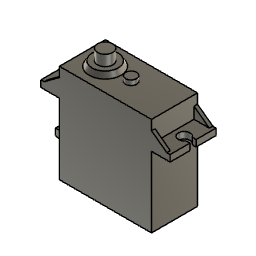
GWSservo v6 (Autodesk Fusion 360 design; units mm, degrees)
Autodesk Fusion 360 part; units mm, degrees
sketch "スケッチ1" plane through (0, 0, 0) normal (0, 1, 0) x (1, 0, 0)
  line L0 (-28.35, -21.75) -> (0, -21.75)
  line L1 (0, -21.75) -> (0, 0)
  line L2 (0, 0) -> (-28.35, 0)
  line L3 (-28.35, 0) -> (-28.35, -21.75)
  dimension "d1" = 28.35
  dimension "d2" = 21.75
  constraint horizontal L0
  constraint vertical L1
  constraint horizontal L2
  constraint vertical L3
  constraint coincident L1.end L2.start
  measures "d1" distance of L0.start L0.end
  measures "d2" distance of L0.start L2.end
extrude "押し出し1" add sketch "スケッチ1" along normal blind 14.15 makes body 1
sketch "スケッチ2" plane through (0, 0, 0) normal (0, -1, 0) x (1, 0, 0)
  line L0 (-28.35, 21.75) -> (-28.35, 0)
  line L1 (-28.35, 0) -> (0, 0)
  line L2 (0, 0) -> (0, 21.75)
  line L3 (0, 21.75) -> (-28.35, 21.75)
  line L4 (-34.075, 21.75) -> (5.725, 21.75)
  line L5 (5.725, 21.75) -> (5.725, 23.75)
  line L6 (0, 27.25) -> (0, 30.25)
  line L7 (0, 30.25) -> (-28.35, 30.25)
  line L8 (-28.35, 30.25) -> (-28.35, 27.25)
  line L9 (-34.075, 23.75) -> (-34.075, 21.75)
  line L10 (-28.35, 27.25) -> (-33.075, 23.75)
  line L11 (-33.075, 23.75) -> (-34.075, 23.75)
  line L12 (0, 27.25) -> (4.725, 23.75)
  line L13 (4.725, 23.75) -> (5.725, 23.75)
  dimension "d5" = 2
  dimension "d6" = 30.25
  dimension "d7" = 5.5
  dimension "d8" = 39.8
  dimension "d9" = 1
  dimension "d15" = 3
  dimension "d16" = 28.35
  dimension "d73" = 28.35
  constraint perpendicular L4 L5
  constraint perpendicular L4 L6
  constraint perpendicular L7 L8
  constraint vertical L9
  constraint midpoint L3 L4
  constraint collinear L3 L4
  constraint equal L5 L9
  constraint equal L6 L8
  constraint vertical L8
  constraint collinear L0 L8
  constraint equal L10 L12
  constraint equal L11 L13
  constraint horizontal L13
  measures "d5" distance of L4.start L9.start
  measures "d6" distance of L1 L7
  measures "d7" distance of L4 L8.end
  measures "d8" distance of L5.end L9.start
  measures "d9" distance of L5.end L12.end
  measures "d15" distance of L6.start L7
  measures "d16" distance of L6.end L7.end
  measures "d73" distance of L0 L2
extrude "押し出し2" add sketch "スケッチ2" against normal blind 14.15 contours L3 L4 L5 L6 L7 L8 L9 L10 L11 L12 L13 bodies 1
ref_plane "作業平面1" through (0, 7.075, 0) normal (0, 1, 0) x (0, 0, 1)
sketch "スケッチ3" plane through (0, 7.075, 0) normal (0, 1, 0) x (1, 0, 0)
  line L0 (0, -27.25) -> (4.725, -23.75)
  line L1 (0, -23.75) -> (0, -27.25)
  line L2 (4.725, -23.75) -> (0, -23.75)
  line L3 (-14.175, -35.735) -> (-14.175, -20.735) construction
  line L4 (-33.075, -23.75) -> (-28.35, -23.75)
  line L5 (-28.35, -27.25) -> (-33.075, -23.75)
  line L6 (-28.35, -23.75) -> (-28.35, -27.25)
  line L7 (-28.35, -21.75) -> (-28.35, 0)
  line L8 (-28.35, 0) -> (0, 0)
  line L9 (0, 0) -> (0, -21.75)
  line L10 (0, -21.75) -> (5.725, -21.75)
  line L11 (5.725, -21.75) -> (5.725, -23.75)
  line L12 (5.725, -23.75) -> (4.725, -23.75)
  line L13 (4.725, -23.75) -> (0, -27.25)
  line L14 (0, -27.25) -> (0, -30.25)
  line L15 (0, -30.25) -> (-28.35, -30.25)
  line L16 (-28.35, -30.25) -> (-28.35, -27.25)
  line L17 (-28.35, -27.25) -> (-33.075, -23.75)
  line L18 (-33.075, -23.75) -> (-34.075, -23.75)
  line L19 (-34.075, -23.75) -> (-34.075, -21.75)
  line L20 (-34.075, -21.75) -> (-28.35, -21.75)
  dimension "d70" = 28.35
  dimension "d71" = 14.175
  dimension "d72" = 2
  constraint coincident L0.end L2.start
  constraint horizontal L2
  constraint vertical L1
  constraint vertical L3
  constraint symmetric L1.start L3 L4.end
  constraint symmetric L0.end L3 L4.start
  constraint symmetric L0.start L3 L5.start
  constraint collinear L1 L14
  constraint coincident L0.start L1.end
  measures "d70" distance of L14.end L15.end
  measures "d71" distance of L3 L15.end
  measures "d72" distance of L2 L10
extrude "押し出し3" cut sketch "スケッチ3" along normal mid plane 12 contours L0 L1 L2 L13 | L4 L5 L6 L17 bodies 1
sketch "スケッチ4" plane through (0, 0, 30.25) normal (0, 0, 1) x (-1, 0, 0)
  line L0 (28.35, 0) -> (0, 0)
  line L1 (0, 0) -> (0, -14.15)
  line L2 (0, -14.15) -> (28.35, -14.15)
  line L3 (28.35, -14.15) -> (28.35, 0)
  circle A0 centre (13.35, -7.075) radius 1.7
  circle A1 centre (21.35, -7.075) radius 4.9
  line L4 (28.35, -7.075) -> (-4.65, -7.075) construction
  dimension "d17" = 3.4
  dimension "d18" = 9.8
  dimension "d19" = 15
  dimension "d20" = 7
  dimension "d75" = 14.15
  dimension "d76" = 7.075
  constraint perpendicular L1 L4
  constraint midpoint L3 L4.start
  constraint coincident A0.centre L4
  constraint coincident A1.centre L4
  measures "d17" diameter of A0
  measures "d18" diameter of A1
  measures "d19" distance of A0.centre L4.start
  measures "d20" distance of A1.centre L4.start
  measures "d75" distance of L0 L2
  measures "d76" distance of L0 A1.centre
extrude "押し出し4" add sketch "スケッチ4" along normal blind 1.5 contours A0 bodies 1
ref_plane "作業平面2" through (-14.175, 7.075, 31.75) normal (0, 0, 1) x (1, 0, 0)
sketch "スケッチ5" plane through (-14, 7, 31.75) normal (0, 0, 1) x (1, 0, 0)
  circle A0 centre (-7.35, 0.075) radius 4
  line L0 (-14.35, -7) -> (-14.35, 7.15)
  line L1 (14, -7) -> (-14.35, -7)
  dimension "d24" = 8
  dimension "d25" = 7
  dimension "d74" = 7.075
  dimension "d77" = 14.15
  measures "d24" diameter of A0
  measures "d25" distance of A0.centre L0
  measures "d74" distance of A0.centre L1
  measures "d77" distance of L0.end L1
loft "ロフト1" add profiles "スケッチ4", "スケッチ5" section 1 contours A1 section 2 bodies 1
sketch "スケッチ6" plane through (0, 0, 31.75) normal (0, 0, 1) x (-1, 0, 0)
  circle A0 centre (21.35, -7.075) radius 4
  circle A1 centre (21.35, -7.075) radius 2.35
  dimension "d26" = 4.7
  constraint concentric A0 A1
  measures "d26" diameter of A1
extrude "押し出し5" add sketch "スケッチ6" along normal blind 3.3 contours A1 bodies 1
sketch "スケッチ7" plane through (0, 0, 0) normal (0, 0, -1) x (1, 0, 0)
  line L0 (0, 0) -> (-28.35, 0)
  line L1 (-28.35, 0) -> (-28.35, -14.15)
  line L2 (-28.35, -14.15) -> (0, -14.15)
  line L3 (0, -14.15) -> (0, 0)
  circle A0 centre (-6.5, -3.5) radius 2.35
  circle A1 centre (-6.5, -10.65) radius 2.35
  dimension "d29" = 3.5
  dimension "d30" = 3.5
  dimension "d31" = 4.7
  dimension "d32" = 4.7
  dimension "d33" = 6.5
  dimension "d34" = 6.5
  measures "d29" distance of L0 A0.centre
  measures "d30" distance of L2 A1.centre
  measures "d31" diameter of A0
  measures "d32" diameter of A1
  measures "d33" distance of L3 A0.centre
  measures "d34" distance of L3 A1.centre
extrude "押し出し6" add sketch "スケッチ7" along normal blind 0.5 contours A0 | A1 bodies 1
sketch "スケッチ8" plane through (-28.35, 0, 0) normal (-1, 0, 0) x (0, -1, 0)
  line L0 (0, 0) -> (0, 21.75)
  line L1 (0, 21.75) -> (-14.15, 21.75)
  line L2 (-14.15, 21.75) -> (-14.15, 0)
  line L3 (-14.15, 0) -> (0, 0)
  line L4 (-10.4, 9.4) -> (-3.75, 9.4)
  line L5 (-3.75, 9.4) -> (-3.75, 5.4)
  line L6 (-3.75, 5.4) -> (-10.4, 5.4)
  line L7 (-10.4, 5.4) -> (-10.4, 9.4)
  dimension "d37" = 3.75
  dimension "d38" = 3.75
  dimension "d39" = 5.4
  dimension "d40" = 4
  constraint horizontal L4
  constraint vertical L5
  constraint horizontal L6
  constraint vertical L7
  measures "d37" distance of L2 L7
  measures "d38" distance of L0 L5
  measures "d39" distance of L3 L6
  measures "d40" distance of L4.start L6.end
extrude "押し出し7" add sketch "スケッチ8" along normal blind 1 contours L4 L5 L6 L7 bodies 1
sketch "スケッチ9" plane through (-29.35, 0, 0) normal (-1, 0, 0) x (0, -1, 0)
  line L0 (-10.4, 5.4) -> (-3.75, 5.4)
  line L1 (-3.75, 5.4) -> (-3.75, 9.4)
  line L2 (-3.75, 9.4) -> (-10.4, 9.4)
  line L3 (-10.4, 9.4) -> (-10.4, 5.4)
  line L4 (-9.9, 8.9) -> (-4.25, 8.9)
  line L5 (-4.25, 8.9) -> (-4.25, 5.9)
  line L6 (-4.25, 5.9) -> (-9.9, 5.9)
  line L7 (-9.9, 5.9) -> (-9.9, 8.9)
  dimension "d43" = 0.5
  dimension "d44" = 0.5
  dimension "d45" = 0.5
  dimension "d46" = 0.5
  constraint horizontal L4
  constraint vertical L5
  constraint horizontal L6
  constraint vertical L7
  measures "d43" distance of L0 L6
  measures "d44" distance of L1 L5
  measures "d45" distance of L2 L4
  measures "d46" distance of L3 L7
ref_plane "作業平面3" through (-34.35, 7.075, 7.4) normal (-1, 0, 0) x (0, -1, 0)
sketch "スケッチ10" plane through (-34.35, 7, 7) normal (-1, 0, 0) x (0, 1, 0)
  line L0 (2.4, -1.4) -> (-2.25, -1.4)
  line L1 (-2.25, -1.4) -> (-2.25, 0.6)
  line L2 (-2.25, 0.6) -> (2.4, 0.6)
  line L3 (2.4, 0.6) -> (2.4, -1.4)
  line L4 (2.9, -1.9) -> (-2.75, -1.9)
  line L5 (2.9, 1.1) -> (2.9, -1.9)
  line L6 (-2.75, 1.1) -> (2.9, 1.1)
  line L7 (-2.75, -1.9) -> (-2.75, 1.1)
  dimension "d48" = 0.5
  dimension "d49" = 0.5
  dimension "d50" = 0.5
  dimension "d51" = 0.5
  constraint horizontal L0
  constraint vertical L1
  constraint horizontal L2
  constraint vertical L3
  measures "d48" distance of L0 L4
  measures "d49" distance of L3 L5
  measures "d50" distance of L2 L6
  measures "d51" distance of L1 L7
loft "ロフト2" add profiles "スケッチ9", "スケッチ10" section 1 contours L4 L5 L6 L7 section 2 contours L0 L1 L2 L3 bodies 1
sketch "スケッチ11" plane through (0, 0, 23.75) normal (0, 0, 1) x (-1, 0, 0)
  line L0 (-5.725, 0) -> (-5.725, -14.15)
  line L1 (-5.725, -14.15) -> (-4.725, -14.15)
  line L2 (-4.725, -14.15) -> (-4.725, -13.075)
  line L3 (-4.725, 0) -> (-5.725, 0)
  line L4 (0, 0) -> (0, -14.15)
  line L5 (-5.725, -6.1244) -> (-4.5285, -6.1244)
  line L6 (-4.5285, -8.0256) -> (-5.725, -8.0256)
  arc A0 (-4.5285, -8.0256) -> (-4.5285, -6.1244) centre (-3, -7.075) ccw
  line L7 (-5.725, -8.0256) -> (-5.725, -6.1244)
  line L8 (14.175, -24.65) -> (14.175, -3.65) construction
  line L9 (34.075, -8.0256) -> (34.075, -6.1244)
  line L10 (32.8785, -8.0256) -> (34.075, -8.0256)
  arc A1 (32.8785, -6.1244) -> (32.8785, -8.0256) centre (31.35, -7.075) ccw
  line L11 (34.075, -6.1244) -> (32.8785, -6.1244)
  line L12 (-3, -7.075) -> (-8.45, -7.075) construction
  line L13 (0, -14.15) -> (-4.725, -14.15) construction
  line L14 (34.075, 0) -> (33.075, 0) construction
  line L15 (33.075, 0) -> (33.075, -1.075) construction
  line L16 (33.075, -14.15) -> (34.075, -14.15) construction
  line L17 (34.075, -14.15) -> (34.075, 0) construction
  line L18 (33.075, 0) -> (28.35, 0) construction
  line L19 (28.35, 0) -> (28.35, -1.075) construction
  line L20 (28.35, -14.15) -> (33.075, -14.15) construction
  line L21 (33.075, -1.075) -> (33.075, 0) construction
  circle A2 centre (21.35, -7.075) radius 4.9 construction
  circle A3 centre (13.35, -7.075) radius 1.7 construction
  line L22 (28.35, 0) -> (0, 0) construction
  line L23 (0, 0) -> (0, -14.15) construction
  line L24 (0, -14.15) -> (28.35, -14.15) construction
  line L25 (28.35, -14.15) -> (28.35, 0) construction
  line L26 (0, 0) -> (-4.725, 0) construction
  line L27 (-4.725, 0) -> (-4.725, -1.075) construction
  line L28 (-4.725, -14.15) -> (0, -14.15) construction
  line L29 (0, -1.075) -> (0, 0) construction
  line L30 (34.075, -14.15) -> (-5.725, -14.15) construction
  line L31 (34.075, -14.15) -> (-5.725, -14.15) construction
  line L32 (-4.725, -13.075) -> (0, -13.075)
  line L33 (0, -13.075) -> (0, -1.075)
  line L34 (0, -1.075) -> (-4.725, -1.075)
  line L35 (-4.725, -1.075) -> (-4.725, 0)
  line L36 (-4.725, -1.075) -> (0, -1.075)
  line L37 (0, -13.075) -> (-4.725, -13.075)
  line L38 (-4.725, -13.075) -> (-4.725, -14.15)
  line L39 (0, -14.15) -> (0, -13.075)
  line L40 (33.075, -1.075) -> (28.35, -1.075)
  line L41 (28.35, -1.075) -> (28.35, -13.075)
  line L42 (28.35, -13.075) -> (33.075, -13.075)
  line L43 (33.075, -13.075) -> (33.075, -14.15)
  line L44 (28.35, -1.075) -> (33.075, -1.075)
  line L45 (33.075, -13.075) -> (28.35, -13.075)
  line L46 (28.35, -13.075) -> (28.35, -14.15)
  line L47 (33.075, -14.15) -> (33.075, -13.075)
  point P0 (-4.65, -7.075)
  dimension "d61" = 3.6
  dimension "d62" = 3
  dimension "d67" = 1.9011
  dimension "d68" = 14.15
  dimension "d69" = 7.075
  constraint horizontal L5
  constraint horizontal L6
  constraint coincident L0 L6.end
  constraint coincident L0 L5.start
  constraint perpendicular L5 L7
  constraint vertical L8
  constraint symmetric L6.start L8 L10.start
  constraint symmetric L5.end L8 A1.start
  constraint symmetric L6.end L8 L9.start
  constraint symmetric L5.start L8 L9.end
  constraint symmetric A0 L8 A1
  constraint coincident A0.centre L12.start
  constraint perpendicular L2 L12
  constraint midpoint L7 L12
  constraint midpoint L0 L12
  constraint coincident L16.end L17.start
  constraint coincident L0.end L1.start
  constraint horizontal L31
  constraint midpoint L8 L31
  measures "d61" diameter of A0
  measures "d62" distance of A0.centre L4
  measures "d67" distance of L5 L6
  measures "d68" distance of L4.start L13
  measures "d69" vertical distance of A0.centre L1.end
extrude "押し出し8" cut sketch "スケッチ11" against normal blind 2 contours L0 L5 L6 A0 L7 | L9 L10 A1 L11 bodies 1
copy_body "ボディ -> コンポーネント1" bodies 1 removing the originals makes body 2 in component "Component"
component "Component" placed x (1, 0, 0) y (0, 1, 0) z (0, 0, 1) at (0, 0, 0)
